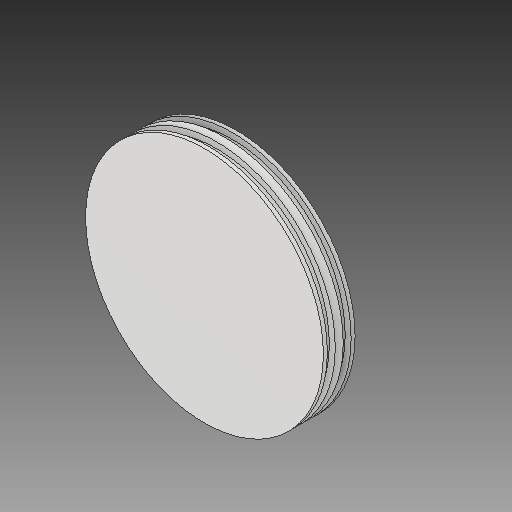
# Autodesk Inventor part: PulleyAdapter
Saved by Autodesk Inventor 2017 (Build 210142000, 142)
## iProperties
Created: 2017-02-11
Part Number: PulleyAdapter
Material: ABS Plastic
Document SubType Name: Modeling
Designer: aribu
Density: 1.06 g/cm^3
Appearance: Smooth - White
Mass: 23.3866 g
Surface Area: 86.2287 cm^2
Volume: 22.0629 cm^3
Author: aribu
Autodesk Inventor part; units mm, degrees
ref_plane "YZ Plane" through (0, 0, 0) normal (1, 0, 0) x (0, 1, 0)
ref_plane "XZ Plane" through (0, 0, 0) normal (0, 1, 0) x (-1, 0, 0)
ref_plane "XY Plane" through (0, 0, 0) normal (0, 0, 1) x (1, 0, 0)
sketch "Sketch3" plane through (0, 0, 0) normal (0, 0, 1) x (1, 0, 0)
  circle A0 centre (0, 0) radius 4.45
  dimension "d11" = 8.9
  constraints: 1 centre point, 1 coincident
  measures "d11" diameter of A0
extrude "Extrusion3" add sketch "Sketch3" along normal blind 6
sketch "Sketch4" plane through (0, 0, 6) normal (0, 0, 1) x (1, 0, 0)
  circle A0 centre (0, 0) radius 30
  dimension "d14" = 60
  constraints: 1 centre point, 1 coincident
  measures "d14" diameter of A0
extrude "Extrusion4" add sketch "Sketch4" along normal blind 8
ref_plane "Work Plane2" through (0, 0, 8) normal (0, 0, 1) x (1, 0, 0)
ref_plane "Work Plane1" through (0, 0, 10) normal (0, 0, 1) x (1, 0, 0)
sketch "Sketch5" plane through (0, 0, 8) normal (0, 0, 1) x (1, 0, 0)
  circle A0 centre (0, 0) radius 28.5
  circle A1 centre (0, 0) radius 30
  dimension "d17" = 57
  dimension "d18" = 60
  constraints: 2 centre point, 2 coincident
  measures "d17" diameter of A0
  measures "d18" diameter of A1
extrude "Extrusion5" cut sketch "Sketch5" along normal mid plane 2
mirror "Mirror1" about plane through (0, 0, 10) normal (0, 0, 1) of "Extrusion5"
sketch "Sketch7" plane through (0, 0, 0) normal (0, 0, -1) x (-1, 0, 0)
  line L0 (-3.4063, 0) -> (1.7033, -2.95)
  line L1 (1.7033, -2.95) -> (1.7033, 2.95)
  line L2 (-3.4063, 0) -> (1.7033, 2.95)
  dimension "d29" = 5.9
  dimension "d30" = 5.9
  dimension "d34" = 5.9
  constraints: 6 end point, 1 vertical
  measures "d29" distance of L0.start L0.end
  measures "d30" distance of L0.end L1.end
  measures "d34" distance of L0.start L1.end
extrude "Extrusion7" add sketch "Sketch7" along normal blind 12
sketch "Sketch8" plane through (-1.7033, -2.95, 0) normal (-1, 0, 0) x (0, 0, 1)
  line L0 (0, 2.95) -> (-12, 2.95) projected
  circle A0 centre (-10.9447, 2.95) radius 0.75
  dimension "d37" = 1.5
  constraints: 1 centre point, 1 point on line
  measures "d37" diameter of A0
extrude "Extrusion8" cut sketch "Sketch8" against normal blind 12
ref_plane "Work Plane3" through (0, 0, 10) normal (0, 0, 1) x (1, 0, 0)
ref_plane "Work Plane4" through (0, 0, 12) normal (0, 0, 1) x (1, 0, 0)
equation "\"d29\" = d34"
equation "\"d30\" = d34"
body "Solid2"
